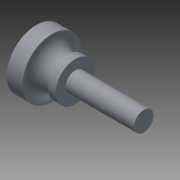
# Autodesk Inventor part: 零件4-4.2
Saved by Autodesk Inventor 2014 (Build 180170000, 170)
## iProperties
Created: 2018-10-26
Part Number: 零件4-4.2
Material: 常规
Document SubType Name: Modeling
Designer: Administrator
Density: 1 g/cm^3
Appearance: 默认
Author: Administrator
Autodesk Inventor part; units mm, degrees
ref_plane "YZ Plane" through (0, 0, 0) normal (1, 0, 0) x (0, 1, 0)
ref_plane "XZ Plane" through (0, 0, 0) normal (0, 1, 0) x (-1, 0, 0)
ref_plane "XY Plane" through (0, 0, 0) normal (0, 0, 1) x (1, 0, 0)
sketch "草图1" plane through (0, 0, 0) normal (0, 0, 1) x (1, 0, 0)
  line L0 (-126.7986, 0) -> (152.2058, 0)
  line L1 (131.579, 0) -> (131.579, 5)
  line L2 (131.579, 5) -> (96.579, 5)
  line L3 (96.579, -20.693) -> (96.579, 5)
  line L4 (96.579, 10) -> (96.579, 5)
  line L5 (92.579, 10) -> (96.579, 10)
  line L6 (92.579, 10) -> (92.579, 0)
  line L7 (84.579, 0) -> (84.579, 15)
  line L8 (84.579, 15) -> (76.579, 15)
  line L9 (76.579, 15) -> (76.579, 0)
  line L10 (91.079, 8.5) -> (92.579, 8.5)
  arc A0 (84.579, 15) -> (91.079, 8.5) centre (91.079, 15) ccw
  point P0 (0, 0)
  dimension "d0" = 6.5
  dimension "d1" = 5
  dimension "d2" = 35
  dimension "d3" = 4
  dimension "d4" = 10
  dimension "d5" = 17
  dimension "d6" = 8
  dimension "d7" = 15
  dimension "d8" = 55
  constraints: 22 end point, 7 perpendicular, 6 point on line, 2 parallel, 2 point on circle, 2 tangent, 1 centre point, 1 collinear, 1 horizontal
  measures "d0" radius of A0
  measures "d1" distance of L1.start L1.end
  measures "d2" distance of L1.end L2.end
  measures "d3" distance of L5.start L4.start
  measures "d4" distance of L5.start L6.end
  measures "d5" diameter of L10 L0
  measures "d6" distance of L7.end L8.end
  measures "d7" distance of L8.end L9.end
  measures "d8" distance between parallel lines of L1 L9
revolve "旋转1" add sketch "草图1" angle 360 about axis through (-126.7986, 0, 0) along (1, 0, 0)
